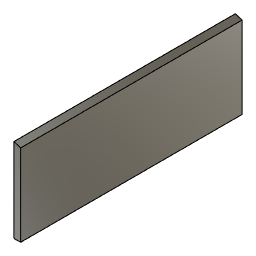
back1-bot v2 (Autodesk Fusion 360 design; units mm, degrees)
Autodesk Fusion 360 part; units mm, degrees
note: some values were not read from the file. Set by a fixed rule: which sketch regions a step uses.
sketch "Esquisse1" plane through (0, 0, 0) normal (0, 1, 0) x (1, 0, 0)
  line L0 (0, 0) -> (4, 0)
  line L1 (4, 0) -> (4, -48.7196)
  line L2 (0, -50) -> (0, 0)
  line L3 (0, -50) -> (4, -48.7196)
  line L4 (0, -50) -> (4.2058, -50) construction
  dimension "d1" = 4
  dimension "d2" = 50
  dimension "d5" = 17.75
  constraint horizontal L0
  constraint vertical L1
  constraint vertical L2
  constraint coincident L0.start L2.end
  constraint horizontal L4
  measures "d1" distance of L0.start L0.end
  measures "d2" distance of L0.start L2.start
  measures "d5" angle of L3 L4
extrude "Extrusion1" add sketch "Esquisse1" along normal blind 132
